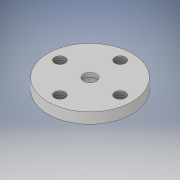
# Autodesk Inventor part: CH
Saved by Autodesk Inventor 2019 (Build 230136000, 136)
## iProperties
Created: 2022-02-24
Part Number: CH
Material: Ogólny
Document SubType Name: Modeling
Designer: Tomasz Krakowski
Density: 1 g/cm^3
Appearance: Domyślna
Author: Tomasz Krakowski
Autodesk Inventor part; units mm, degrees
note: some values were not read from the file. Chosen so that the rebuilt part matches the saved one: direction of "Hole1".
ref_plane "YZ Plane" through (0, 0, 0) normal (1, 0, 0) x (0, 1, 0)
ref_plane "XZ Plane" through (0, 0, 0) normal (0, 1, 0) x (-1, 0, 0)
ref_plane "XY Plane" through (0, 0, 0) normal (0, 0, 1) x (1, 0, 0)
sketch "Sketch1" plane through (0, 0, 0) normal (0, 1, 0) x (-1, 0, 0)
  circle A0 centre (0, 0) radius 9.75
  circle A1 centre (0, 0) radius 1.5
  circle A2 centre (0, 0) radius 7 construction
  line L0 (0, 0) -> (7, 0) construction
  point P0 (0, 7)
  point P1 (-7, 0)
  point P2 (0, -7)
  dimension "d3" = 14
  dimension "d0" = 19.5
  dimension "d1" = 3
  dimension "d16" = 360
  constraints: 4 coincident, 2 centre point, 2 end point, 1 horizontal, 1 horizontal alignment, 7 other
  measures "d0" diameter of A0
  measures "d1" diameter of A1
extrude "Extrusion1" add sketch "Sketch1" along normal blind 2.5
sketch "Sketch2" plane through (0, 0, 0) normal (0, -1, 0) x (1, 0, 0)
  circle A0 centre (0, 0) radius 4.375
  circle A1 centre (0, 0) radius 3
  dimension "d10" = 8.75
  dimension "d11" = 6
  constraints: 2 centre point, 2 coincident
  measures "d10" diameter of A0
  measures "d11" diameter of A1
extrude "Extrusion2" add sketch "Sketch2" along normal blind 2.5
sketch "Sketch3" plane through (0, 0, 0) normal (0, -1, 0) x (1, 0, 0)
  circle A0 centre (0, 0) radius 3 projected
  circle A1 centre (0, 0) radius 1.5 projected
extrude "Extrusion3" cut sketch "Sketch3" against normal blind 1.5
sketch "Sketch4" plane through (0, 2.5, 0) normal (0, 1, 0) x (1, 0, 0)
  circle A0 centre (0, 0) radius 7 construction
  line L0 (0, 7) -> (0, 0) construction
  point P0 (-7, 0)
  point P1 (0, -7)
  point P2 (7, 0)
  dimension "d20" = 14
  dimension "d23" = 360
  constraints: 2 end point, 1 coincident, 1 vertical, 1 vertical alignment, 7 other
hole "Hole1" at (-7, 2.5, 0) at (0, 2.5, 7) at (7, 2.5, 0) at (0, 2.5, -7) direction (0, -1, 0) diameter 2.459 end up to surface thread size "M3x0.5" class "6H" standard "ISO Metric profile"
body "Solid1"
